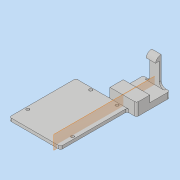
# Autodesk Inventor part: arduinomount
Saved by Autodesk Inventor 2017 (Build 210142000, 142)
## iProperties
Created: 2017-02-25
Part Number: arduinomount
Material: Generic
Document SubType Name: Modeling
Designer: Joshua Yuan
Density: 1 g/cm^3
Appearance: Default
Author: Joshua Yuan
Autodesk Inventor part; units mm, degrees
ref_plane "YZ Plane" through (0, 0, 0) normal (1, 0, 0) x (0, 1, 0)
ref_plane "XZ Plane" through (0, 0, 0) normal (0, 1, 0) x (-1, 0, 0)
ref_plane "XY Plane" through (0, 0, 0) normal (0, 0, 1) x (1, 0, 0)
sketch "Sketch1" plane through (0, 0, 0) normal (0, 1, 0) x (-1, 0, 0)
  line L0 (13.8213, 11.9209) -> (-36.1787, 11.9209)
  line L1 (-38.1787, 9.9209) -> (-38.1787, -58.0791)
  line L2 (-38.1787, -58.0791) -> (13.8213, -58.0791)
  line L3 (15.8213, -56.0791) -> (15.8213, 9.9209)
  line L4 (-20.1787, -58.0791) -> (-48.1787, -58.0791)
  line L5 (-48.1787, -58.0791) -> (-48.1787, -93.0791)
  line L6 (-48.1787, -93.0791) -> (-20.1787, -93.0791)
  line L7 (-20.1787, -93.0791) -> (-20.1787, -58.0791)
  arc A0 (15.8213, 9.9209) -> (13.8213, 11.9209) centre (13.8213, 9.9209) ccw
  arc A1 (13.8213, -58.0791) -> (15.8213, -56.0791) centre (13.8213, -56.0791) ccw
  arc A2 (-36.1787, 11.9209) -> (-38.1787, 9.9209) centre (-36.1787, 9.9209) ccw
  point P0 (0, 0)
  point P1 (15.8213, 11.9209)
  point P2 (-38.1787, 11.9209)
  point P3 (15.8213, -58.0791)
  dimension "d0" = 54
  dimension "d1" = 70
  dimension "d2" = 28
  dimension "d3" = 10
  dimension "d4" = 35
  dimension "d20" = 2
  constraints: 16 end point, 7 point on line, 6 point on circle, 6 tangent, 4 parallel, 3 centre point, 2 equal radius, 2 horizontal, 2 perpendicular
  measures "d0" distance of point (15.821, 11.921) point (-38.179, 11.921)
  measures "d1" distance of point (-38.179, 11.921) L1.end
  measures "d2" distance of L5.end L6.end
  measures "d3" distance between parallel lines of L1 L5
  measures "d4" distance of L4.end L5.end
  measures "d20" radius of A0
extrude "Extrusion1" add sketch "Sketch1" against normal blind 3.175
sketch "Sketch2" plane through (0, 0, 0) normal (0, 1, 0) x (1, 0, 0)
  line L0 (20.1787, 93.0791) -> (20.1787, 58.0791) projected
  line L1 (48.1787, 58.0791) -> (48.1787, 93.0791) projected
  line L2 (20.1787, 93.0791) -> (48.1787, 93.0791)
  line L3 (48.1787, 93.0791) -> (48.1787, 72.0791)
  line L4 (48.1787, 72.0791) -> (20.1787, 72.0791)
  line L5 (20.1787, 72.0791) -> (20.1787, 93.0791)
  line L6 (38.1787, 58.0791) -> (48.1787, 58.0791) projected
  point P0 (0, 0)
  dimension "d7" = 14
  constraints: 8 end point, 2 parallel, 1 horizontal, 1 perpendicular, 1 point on line
  measures "d7" distance between parallel lines of L6 L4
extrude "Extrusion2" add sketch "Sketch2" along normal blind 3
sketch "Sketch3" plane through (0, 0, 0) normal (0, 1, 0) x (1, 0, 0)
  line L0 (48.1787, 72.0791) -> (20.1787, 72.0791) projected
  line L1 (48.1787, 93.0791) -> (48.1787, 58.0791) projected
  line L2 (20.1787, 72.0791) -> (48.1787, 72.0791)
  line L3 (48.1787, 72.0791) -> (48.1787, 58.0791)
  line L4 (48.1787, 58.0791) -> (20.1787, 58.0791)
  line L5 (20.1787, 58.0791) -> (20.1787, 72.0791)
  point P0 (0, 0)
  constraints: 8 end point, 2 parallel, 1 horizontal, 1 perpendicular
extrude "Extrusion3" add sketch "Sketch3" along normal blind 10
ref_plane "Work Plane1" through (34.1787, -3.175, -58.0791) normal (1, 0, 0) x (0, 0, -1)
sketch "Sketch4" plane through (34.1787, -3.175, -58.0791) normal (1, 0, 0) x (0, 0, -1)
  line L0 (29, 30.175) -> (33, 30.175)
  line L1 (33, 30.175) -> (33, 6.175)
  line L2 (35, 6.175) -> (14, 6.175) projected
  line L3 (35, 6.175) -> (35, 35.175)
  arc A0 (35, 35.175) -> (29, 30.175) centre (35, 29.075) ccw
  point P0 (-58.0791, 3.175)
  dimension "d12" = 2
  dimension "d13" = 29
  dimension "d14" = 24
  dimension "d15" = 4
  constraints: 6 end point, 2 point on circle, 2 point on line, 1 centre point, 1 horizontal, 1 perpendicular, 1 vertical
  measures "d12" distance between parallel lines of L3 L1
  measures "d13" distance of L2.start L3.end
  measures "d14" distance of L0.end L1.end
  measures "d15" distance of L0.start L0.end
extrude "Extrusion4" add sketch "Sketch4" along normal mid plane 10
sketch "Sketch5" plane through (0, 0, 0) normal (0, 1, 0) x (1, 0, 0)
  line L0 (37.8591, -10.4638) -> (37.8591, 55.5762)
  line L1 (37.8591, 55.5762) -> (35.3191, 55.5762)
  line L2 (35.3191, 55.5762) -> (32.7791, 58.1162)
  line L3 (32.7791, 58.1162) -> (-0.2409, 58.1162)
  line L4 (-0.2409, 58.1162) -> (-2.7809, 55.5762)
  line L5 (-2.7809, 55.5762) -> (-14.2109, 55.5762)
  line L6 (-14.2109, 55.5762) -> (-15.4809, 54.3062)
  line L7 (-15.4809, 54.3062) -> (-15.4809, -10.4638)
  line L8 (-15.4809, -10.4638) -> (37.8591, -10.4638)
  spline S0 degree 3 poles (30.2391, 57.1613) (31.1145, 57.1613) (31.8242, 56.4516) (31.8242, 55.5762) (31.8242, 54.7008) (31.1145, 53.9911) (30.2391, 53.9911) (29.3637, 53.9911) (28.654, 54.7008) (28.654, 55.5762) (28.654, 56.4516) (29.3637, 57.1613) (30.2391, 57.1613) knots 0 0 0 0 1 1 1 2 2 2 3 3 3 4 4 4 4
  line L9 (30.2391, 57.1613) -> (31.1145, 57.1613) construction
  line L10 (31.1145, 57.1613) -> (31.8242, 56.4516) construction
  line L11 (31.8242, 56.4516) -> (31.8242, 55.5762) construction
  line L12 (31.8242, 55.5762) -> (31.8242, 54.7008) construction
  line L13 (31.8242, 54.7008) -> (31.1145, 53.9911) construction
  line L14 (31.1145, 53.9911) -> (30.2391, 53.9911) construction
  line L15 (30.2391, 53.9911) -> (29.3637, 53.9911) construction
  line L16 (29.3637, 53.9911) -> (28.654, 54.7008) construction
  line L17 (28.654, 54.7008) -> (28.654, 55.5762) construction
  line L18 (28.654, 55.5762) -> (28.654, 56.4516) construction
  line L19 (28.654, 56.4516) -> (29.3637, 57.1613) construction
  line L20 (29.3637, 57.1613) -> (30.2391, 57.1613) construction
  spline S1 degree 3 poles (2.2991, 57.1613) (3.1745, 57.1613) (3.8842, 56.4516) (3.8842, 55.5762) (3.8842, 54.7008) (3.1745, 53.9911) (2.2991, 53.9911) (1.4237, 53.9911) (0.714, 54.7008) (0.714, 55.5762) (0.714, 56.4516) (1.4237, 57.1613) (2.2991, 57.1613) knots 0 0 0 0 1 1 1 2 2 2 3 3 3 4 4 4 4
  line L21 (2.2991, 57.1613) -> (3.1745, 57.1613) construction
  line L22 (3.1745, 57.1613) -> (3.8842, 56.4516) construction
  line L23 (3.8842, 56.4516) -> (3.8842, 55.5762) construction
  line L24 (3.8842, 55.5762) -> (3.8842, 54.7008) construction
  line L25 (3.8842, 54.7008) -> (3.1745, 53.9911) construction
  line L26 (3.1745, 53.9911) -> (2.2991, 53.9911) construction
  line L27 (2.2991, 53.9911) -> (1.4237, 53.9911) construction
  line L28 (1.4237, 53.9911) -> (0.714, 54.7008) construction
  line L29 (0.714, 54.7008) -> (0.714, 55.5762) construction
  line L30 (0.714, 55.5762) -> (0.714, 56.4516) construction
  line L31 (0.714, 56.4516) -> (1.4237, 57.1613) construction
  line L32 (1.4237, 57.1613) -> (2.2991, 57.1613) construction
  spline S2 degree 3 poles (-12.9409, 6.3613) (-12.0655, 6.3613) (-11.3558, 5.6516) (-11.3558, 4.7762) (-11.3558, 3.9008) (-12.0655, 3.1911) (-12.9409, 3.1911) (-13.8163, 3.1911) (-14.526, 3.9008) (-14.526, 4.7762) (-14.526, 5.6516) (-13.8163, 6.3613) (-12.9409, 6.3613) knots 0 0 0 0 1 1 1 2 2 2 3 3 3 4 4 4 4
  line L33 (-12.9409, 6.3613) -> (-12.0655, 6.3613) construction
  line L34 (-12.0655, 6.3613) -> (-11.3558, 5.6516) construction
  line L35 (-11.3558, 5.6516) -> (-11.3558, 4.7762) construction
  line L36 (-11.3558, 4.7762) -> (-11.3558, 3.9008) construction
  line L37 (-11.3558, 3.9008) -> (-12.0655, 3.1911) construction
  line L38 (-12.0655, 3.1911) -> (-12.9409, 3.1911) construction
  line L39 (-12.9409, 3.1911) -> (-13.8163, 3.1911) construction
  line L40 (-13.8163, 3.1911) -> (-14.526, 3.9008) construction
  line L41 (-14.526, 3.9008) -> (-14.526, 4.7762) construction
  line L42 (-14.526, 4.7762) -> (-14.526, 5.6516) construction
  line L43 (-14.526, 5.6516) -> (-13.8163, 6.3613) construction
  line L44 (-13.8163, 6.3613) -> (-12.9409, 6.3613) construction
  spline S3 degree 3 poles (35.3191, 5.0913) (36.1945, 5.0913) (36.9042, 4.3816) (36.9042, 3.5062) (36.9042, 2.6308) (36.1945, 1.9211) (35.3191, 1.9211) (34.4437, 1.9211) (33.734, 2.6308) (33.734, 3.5062) (33.734, 4.3816) (34.4437, 5.0913) (35.3191, 5.0913) knots 0 0 0 0 1 1 1 2 2 2 3 3 3 4 4 4 4
  line L45 (35.3191, 5.0913) -> (36.1945, 5.0913) construction
  line L46 (36.1945, 5.0913) -> (36.9042, 4.3816) construction
  line L47 (36.9042, 4.3816) -> (36.9042, 3.5062) construction
  line L48 (36.9042, 3.5062) -> (36.9042, 2.6308) construction
  line L49 (36.9042, 2.6308) -> (36.1945, 1.9211) construction
  line L50 (36.1945, 1.9211) -> (35.3191, 1.9211) construction
  line L51 (35.3191, 1.9211) -> (34.4437, 1.9211) construction
  line L52 (34.4437, 1.9211) -> (33.734, 2.6308) construction
  line L53 (33.734, 2.6308) -> (33.734, 3.5062) construction
  line L54 (33.734, 3.5062) -> (33.734, 4.3816) construction
  line L55 (33.734, 4.3816) -> (34.4437, 5.0913) construction
  line L56 (34.4437, 5.0913) -> (35.3191, 5.0913) construction
  point P0 (0, 0)
  constraints: 18 end point, 8 other
extrude "Extrusion5" cut sketch "Sketch5" against normal blind 10 contours S0 | S1 | S2 | S3
fillet "Fillet1" radius 2 5 edges at (48.1787, -0.0875, -93.0791) (20.1787, -0.0875, -93.0791) (48.1787, 3.4125, -58.0791) (38.1787, -1.5875, -58.0791) (20.1787, -1.5875, -58.0791)
fillet "Fillet2" radius 5 2 edges at (39.1787, 3, -92.0791) (29.1787, 3, -92.0791)
body "Solid1"
